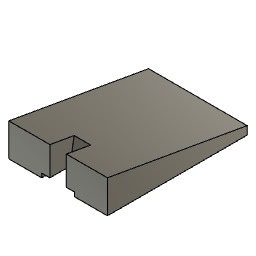
CHEVY_SERVO_HOLDER V3 (Autodesk Fusion 360 design; units mm, degrees)
Autodesk Fusion 360 part; units mm, degrees
sketch "Sketch1" plane through (0, 0, 0) normal (0, 0, 1) x (1, 0, 0)
  line L0 (0, 0) -> (24, 0)
  line L1 (24, 0) -> (24, 34)
  line L2 (24, 34) -> (0, 34)
  line L3 (0, 34) -> (0, 0)
  line L4 (8, 34) -> (8, 0)
  line L5 (16, 34) -> (16, 0)
  dimension "d3" = 34
  dimension "d4" = 24
  dimension "d5" = 8
  dimension "d6" = 8
  constraint horizontal L0
  constraint vertical L1
  constraint horizontal L2
  constraint vertical L3
  constraint coincident L0.start L3.end
  constraint coincident L2 L4.start
  constraint coincident L0 L4.end
  constraint perpendicular L0 L4
  constraint coincident L2 L5.start
  constraint coincident L0 L5.end
  constraint perpendicular L0 L5
  measures "d3" distance of L0.end L1.end
  measures "d4" distance of L1.end L2.end
  measures "d5" distance of L3 L4
  measures "d6" distance of L1 L5
extrude "Extrude1" add sketch "Sketch1" along normal blind 1 contours L0 L2 L3 L4 | L0 L1 L2 L5 makes body 1 at (2.6667, 22.6667, 0) makes body 2 at (18.6667, 22.6667, 0)
sketch "Sketch2" plane through (0, 0, 0) normal (-1, 0, 0) x (0, -1, 0)
  line L0 (-34, 0) -> (0, 0)
  line L1 (0, 0) -> (0, 1)
  line L2 (0, 1) -> (-34, 1)
  line L3 (-34, 1) -> (-34, 0)
  line L4 (0, 1) -> (0, 8)
  line L5 (-34, 1) -> (-34, 2)
  line L6 (0, 8) -> (-34, 2)
  dimension "d9" = 7
  dimension "d12" = 1
  constraint coincident L1.end L2.start
  constraint perpendicular L2 L4
  constraint coincident L2.end L3.start
  constraint perpendicular L2 L5
  measures "d9" distance of L1.end L4.end
  measures "d12" distance of L2.end L5.end
extrude "Extrude3" add sketch "Sketch2" against normal up to surface (24 mm away) contours L2 L4 L5 L6 bodies 1 2
sketch "Sketch3" plane through (0, 1.3691, 7.7584) normal (0, 0.173785, 0.984784) x (-1, 0, 0)
  line L0 (-24, 1.3903) -> (-24, -33.1351)
  line L1 (-24, -33.1351) -> (0, -33.1351)
  line L2 (0, -33.1351) -> (0, 1.3903)
  line L3 (0, 1.3903) -> (-24, 1.3903)
  line L4 (-10, 1.3903) -> (-14, 1.3903)
  line L5 (-14, 1.3903) -> (-14, -4.6097)
  line L6 (-14, -4.6097) -> (-10, -4.6097)
  line L7 (-10, -4.6097) -> (-10, 1.3903)
  dimension "d15" = 4
  dimension "d16" = 6
  constraint horizontal L4
  constraint vertical L5
  constraint horizontal L6
  constraint vertical L7
  constraint midpoint L3 L4
  measures "d15" distance of L4.start L4.end
  measures "d16" distance of L4.end L5.end
extrude "Extrude4" cut sketch "Sketch3" along normal up to surface contours L3 L4 L5 L6 L7 end surface through (0, 0, 1) normal (0, 0, -1) offset 0 bodies 1
equation "Hoogte_SERVO = 34 mm" comment "Hoogte_SERVO"
equation "Breedte_SERVO = 24 mm" comment "Breedte_SERVO"
equation "d3 = Hoogte_SERVO"
equation "d4 = Breedte_SERVO"
equation "d6 = d5"
equation "d9 = 4 mm + 3 mm"
